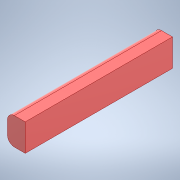
# Autodesk Inventor part: Bumper
Saved by Autodesk Inventor 2020 (Build 240168000, 168)
## iProperties
Created: 2020-01-28
Part Number: Bumper
Material: Generic
Document SubType Name: Modeling
Designer: 1jyng
Density: 1 g/cm^3
Appearance: Smooth - Red
Author: 1jyng
Autodesk Inventor part; units mm, degrees
ref_plane "YZ Plane" through (0, 0, 0) normal (1, 0, 0) x (0, 1, 0)
ref_plane "XZ Plane" through (0, 0, 0) normal (0, 1, 0) x (-1, 0, 0)
ref_plane "XY Plane" through (0, 0, 0) normal (0, 0, 1) x (1, 0, 0)
sketch "Sketch1" plane through (0, 0, 0) normal (0, 0, 1) x (1, 0, 0)
  line L0 (0, 0) -> (-82.55, 0)
  line L1 (-82.55, 0) -> (-82.55, 127)
  line L2 (-82.55, 127) -> (0, 127)
  line L3 (0, 127) -> (0, 0)
  dimension "d0" = 82.55
  dimension "d1" = 127
  constraints: 8 end point, 2 parallel, 1 horizontal, 1 perpendicular
  measures "d0" distance of L1.end L2.end
  measures "d1" distance of L2.end L0.start
extrude "Extrusion1" add sketch "Sketch1" along normal blind 685.8
fillet "Fillet1" radius 31.75 2 edges at (-82.55, 127, 342.9) (-82.55, 0, 342.9)
body "Solid1"
